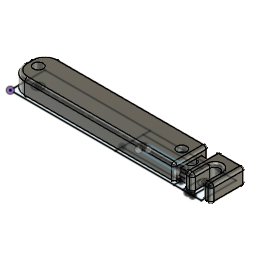
echelon connect sport (Autodesk Fusion 360 design; units mm, degrees)
Autodesk Fusion 360 part; units mm, degrees
note: some values were not read from the file. Set by a fixed rule: which face or edge a step refers to.
sketch "Sketch1" plane through (0, 0, 0) normal (0, 0, 1) x (1, 0, 0)
  line L0 (0, 0) -> (85, 0)
  line L1 (85, 0) -> (85, 18)
  line L2 (85, 18) -> (0, 18)
  line L3 (0, 18) -> (0, 0)
  line L4 (0, 9) -> (85, 9)
  circle A0 centre (5.5, 9) radius 2.525
  line L5 (54.5, 18) -> (54.5, 9)
  line L6 (54.5, 0) -> (54.5, 9)
  circle A1 centre (60, 9) radius 2.5
  circle A2 centre (80, 9) radius 2.5
  line L7 (54.5, 14.5) -> (85, 14.5)
  line L8 (54.5, 3.5) -> (85, 3.5)
  line L9 (60, 11.5) -> (60, 6.5) construction
  line L10 (80, 11.5) -> (80, 6.5) construction
  line L11 (60, 11.5) -> (80, 11.5)
  line L12 (60, 6.5) -> (80, 6.5)
  line L13 (85, 9) -> (62.5333, 9)
  circle A3 centre (92.075, 9) radius 2.575
  line L14 (92.075, 9) -> (92.075, 18) construction
  line L15 (92.075, 9) -> (92.075, 0) construction
  line L16 (85, 0) -> (92.075, 0)
  line L17 (89.5, 9) -> (89.5, 0)
  line L18 (85, 18) -> (92.075, 18)
  line L19 (99.15, 18) -> (92.075, 18)
  line L20 (94.65, 9) -> (94.65, 0)
  line L21 (99.15, 0) -> (92.075, 0)
  line L22 (99.15, 0) -> (99.15, 18)
  dimension "d1" = 85
  dimension "d2" = 18
  dimension "d5" = 5.05
  dimension "d6" = 5.5
  dimension "d8" = 5
  dimension "d10" = 5
  dimension "d11" = 5
  dimension "d12" = 3.5
  dimension "d35" = 20
  dimension "d36" = 5.5
  dimension "d53" = 5.15
  dimension "d54" = 7.075
  constraint horizontal L0
  constraint vertical L1
  constraint horizontal L2
  constraint vertical L3
  constraint coincident L0.start L3.end
  constraint midpoint L3 L4.start
  constraint midpoint L1 L4.end
  constraint coincident L4 A0.centre
  constraint coincident L2 L5.start
  constraint coincident L4 L5.end
  constraint perpendicular L4 L5
  constraint coincident L0 L6.start
  constraint perpendicular L4 L6
  constraint coincident L4 A1.centre
  constraint coincident L4 A2.centre
  constraint coincident L5 L7.start
  constraint coincident L1 L7.end
  constraint perpendicular L1 L7
  constraint symmetric L4 L7.start L8.start
  constraint symmetric L4 L7.end L8.end
  constraint coincident A1 L9.start
  constraint coincident A1 L9.end
  constraint perpendicular L4 L9
  constraint coincident A2 L10.start
  constraint coincident A2 L10.end
  constraint perpendicular L4 L10
  constraint tangent A2 L11
  constraint symmetric L4 L9.start L9.end
  constraint symmetric L4 L10.start L10.end
  constraint perpendicular L1 L13
  constraint coincident L13 A3.centre
  constraint coincident A3.centre L14.start
  constraint perpendicular L2 L14
  constraint perpendicular L0 L15
  constraint perpendicular L15 L16
  constraint coincident A3 L17.start
  constraint coincident L13 L17.start
  constraint coincident L16 L17.end
  constraint tangent A3 L17
  constraint perpendicular L14 L18
  constraint symmetric L0.end L14 L21.start
  constraint symmetric L1.end L14 L19.start
  constraint symmetric L18.end L14 L19.end
  constraint symmetric L14 L15.end L16.end
  constraint symmetric L14 L17.start L20.start
  constraint symmetric L14 L17.end L20.end
  measures "d1" distance of L0.start L0.end
  measures "d2" distance of L0.start L2.end
  measures "d5" diameter of A0
  measures "d6" distance of L4.start A0.centre
  measures "d8" diameter of A1
  measures "d10" diameter of A2
  measures "d11" distance of L1 A2.centre
  measures "d12" distance of L2 L7
  measures "d35" distance of A1.centre A2.centre
  measures "d36" distance of L6 A1.centre
  measures "d53" diameter of A3
  measures "d54" distance of L4.end A3.centre
extrude "Extrude1" add sketch "Sketch1" along normal blind 9.1 contours L0 L3 L4 A0 L6 | L0 L1 L6 L8 | L2 L3 L4 A0 L5 | L1 L4 L6 A1 A2 L8 L12 L13 | L1 L4 L5 A1 A2 L7 L11 L13 | L1 L2 L5 L7 | L4 A1 | L4 A1 | L4 A1 A2 L11 L13 | L4 A1 A2 L12 L13 makes body 1
extrude "Extrude2" cut sketch "Sketch1" along normal blind 6 contours L1 L4 L6 A1 A2 L8 L12 L13 | L1 L4 L5 A1 A2 L7 L11 L13 | L4 A1 | L4 A1 | L4 A1 A2 L11 L13 | L4 A1 A2 L12 L13 bodies 1
extrude "Extrude3" add sketch "Sketch1" along normal blind 5.8 separate body contours L1 L4 L6 A1 A2 L8 L12 L13 | L1 L4 L5 A1 A2 L7 L11 L13 makes body 2
sketch "Sketch3" plane through (54.5, 0, 0) normal (1, 0, 0) x (0, 1, 0)
  line L0 (3.5, 0) -> (14.5, 0)
  line L1 (14.5, 0) -> (14.5, 6)
  line L2 (14.5, 6) -> (3.5, 6)
  line L3 (3.5, 6) -> (3.5, 0)
  line L4 (3.5, 3) -> (2.5, 3) construction
  line L5 (2.5, 3) -> (3.5, 4)
  line L6 (2.5, 3) -> (3.9142, 3) construction
  line L7 (2.5, 3) -> (3.5, 2)
  line L8 (9, 6) -> (9, 0)
  line L9 (15.5, 3) -> (14.5, 4)
  line L10 (15.5, 3) -> (14.5, 2)
  line L11 (15.3586, 3) -> (14.4293, 3.9293)
  line L12 (15.3586, 3) -> (14.4293, 2.0707)
  line L13 (2.6414, 3) -> (3.5707, 2.0707)
  line L14 (2.6414, 3) -> (3.5707, 3.9293)
  dimension "d37" = 1
  dimension "d38" = 45
  dimension "d43" = -0.1
  constraint midpoint L3 L4.start
  constraint perpendicular L3 L4
  constraint horizontal L6
  constraint coincident L3 L5.end
  constraint coincident L3 L7.end
  constraint perpendicular L5 L7
  constraint midpoint L2 L8.start
  constraint midpoint L0 L8.end
  constraint symmetric L4.end L8 L9.start
  constraint symmetric L5.end L8 L9.end
  constraint symmetric L7.end L8 L10.end
  constraint symmetric L8 L11.start L13.start
  constraint symmetric L8 L11.end L14.end
  constraint symmetric L8 L12.end L13.end
  measures "d37" distance of L4.start L4.end
  measures "d38" angle of L5 L6
extrude "Extrude7" cut sketch "Sketch3" along normal up to surface (30.5 mm away) contours L3 L5 L7 L13 L14 | L3 L13 L14 | L1 L9 L10 L11 L12 | L1 L11 L12 bodies 1
extrude "Extrude8" add sketch "Sketch3" along normal up to surface (30.5 mm away) contours L3 L13 L14 | L1 L11 L12 bodies 2
move_face "OffsetFaces1" offset -0.15 4 faces at (74.8333, 14.5, 5.1529) (64.6667, 14.5, 0.7138) (64.6667, 3.5, 0.7138) (74.8333, 3.5, 5.1529) on bodies 2
extrude "Extrude6" add sketch "Sketch1" along normal blind 9.1 contours L1 A3 L16 L17 L18 L19 L20 L21 L22 bodies 2
move_body "Move1" bodies 2 to x (1, 0, 0) y (0, 1, 0) z (0, 0, 1) at (5, 0, 0)
fillet "Fillet2" radius 7.5 2 edges at (0, 18, 4.55) (0, 0, 4.55) on bodies 1 2
fillet "Fillet2" radius 1.5 3 edges at (85, 1.75, 0) (85, 16.25, 0) (85, 9, 9.1) 2 faces at (28.3333, 0, 3.0333) (28.3333, 18, 6.0667) on bodies 1 2
fillet "Fillet2" radius 1.5 2 edges at (0, 9, 9.1) (0, 9, 0) on bodies 1 2
fillet "Fillet2" radius 1.5 5 edges at (90, 1.825, 0) (90, 16.175, 0) (94.5, 4.5, 0) (97.075, 11.575, 0) (99.65, 4.5, 0) 5 faces at (97.1391, 15.8559, 9.1) (91.5, 0, 6.0667) (102.65, 0, 3.0333) (104.15, 6, 3.0333) (94.7167, 18, 3.0333) on bodies 1 2
equation "d54 = 4.5 mm + ( 5.15 / 2 ) * 1 mm"
